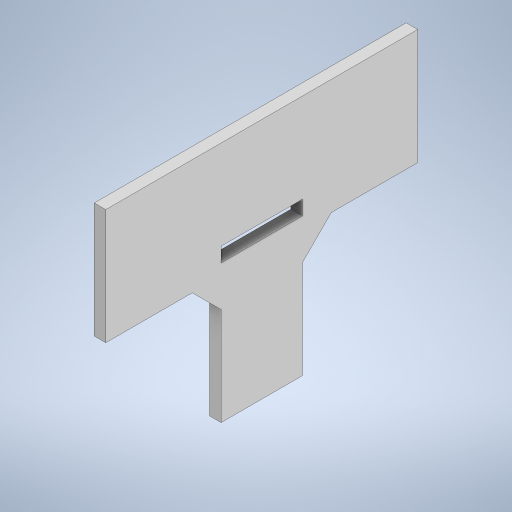
# Autodesk Inventor part: manual_locker_upper_raw
Saved by Autodesk Inventor 2024 (Build 280153000, 153)
## iProperties
Created: 2025-12-30
Part Number: manual_locker_upper_raw
Material: Generic
Document SubType Name: Modeling
Designer: schar
Density: 1 g/cm^3
Appearance: Default
Author: schar
Autodesk Inventor part; units mm, degrees
ref_plane "YZ Plane" through (0, 0, 0) normal (1, 0, 0) x (0, 1, 0)
ref_plane "XZ Plane" through (0, 0, 0) normal (0, 1, 0) x (-1, 0, 0)
ref_plane "XY Plane" through (0, 0, 0) normal (0, 0, 1) x (1, 0, 0)
sketch "Sketch1" plane through (0, 0, 0) normal (1, 0, 0) x (0, 1, 0)
  line L0 (20, 27.056) -> (0, 27.056)
  line L1 (0, 27.056) -> (0, -27.056)
  line L2 (0, -27.056) -> (20, -27.056)
  line L3 (20, -27.056) -> (20, 27.056)
  line L4 (0, 27.056) -> (0, 0)
  line L5 (0, 0) -> (0, -7.056)
  line L6 (0, -7.056) -> (-22, -7.056)
  line L7 (-22, -7.056) -> (-22, 7.056)
  line L8 (-22, 7.056) -> (0, 7.056)
  line L9 (0, 7.056) -> (0, -7.056)
  line L10 (0, 7.056) -> (2, 7.056)
  line L11 (2, 7.056) -> (4.5, 7.056)
  line L12 (4.5, 7.056) -> (4.5, -7.056)
  line L13 (4.5, -7.056) -> (2, -7.056)
  line L14 (2, -7.056) -> (2, 7.056)
  line L15 (0, 7.056) -> (0, 12.056)
  line L16 (0, 12.056) -> (-5, 7.056)
  line L17 (0, -7.056) -> (-5, -7.056)
  line L18 (-5, -7.056) -> (0, -12.056)
  line L19 (0, -7.056) -> (0, -12.056)
  point P0 (0, 0)
  dimension "d0" = 20
  dimension "d1" = 54.112
  dimension "d2" = 27.056
  dimension "d3" = 7.056
  dimension "d4" = 22
  dimension "d5" = 14.112
  dimension "d6" = 2
  dimension "d7" = 2.5
  dimension "d8" = 5
  dimension "d9" = 45
  dimension "d10" = 5
  constraints: 40 end point, 6 parallel, 5 point on line, 4 horizontal, 4 perpendicular, 1 midpoint
  measures "d0" distance of L3.start L1.end
  measures "d1" distance of L1.end L1.start
  measures "d2" distance of L1.start L5.start
  measures "d3" distance of L5.start L5.end
  measures "d4" distance of L8.start L8.end
  measures "d5" distance of L6.end L8.start
  measures "d6" distance of L8.end L10.end
  measures "d7" distance of L12.end L14.start
  measures "d8" distance of L8.end L16.start
  measures "d9" angle of L16 L15
  measures "d10" distance of L5.end L17.end
extrude "Extrusion1" add sketch "Sketch1" along normal blind 2
body "Solid1"
